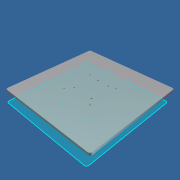
# Autodesk Inventor part: Acrylic_6_Base
Saved by Autodesk Inventor 2012 (Build 160160000, 160)
## iProperties
Created: 2014-03-30
Part Number: Acrylic_6_Base
Material: Default
Document SubType Name: Modeling
Designer: Admin
Density: 1 g/cm^3
Author: Admin
Autodesk Inventor part; units mm, degrees
ref_plane "YZ Plane" through (0, 0, 0) normal (1, 0, 0) x (0, 1, 0)
ref_plane "XZ Plane" through (0, 0, 0) normal (0, 1, 0) x (-1, 0, 0)
ref_plane "XY Plane" through (0, 0, 0) normal (0, 0, 1) x (1, 0, 0)
sketch "Sketch1" plane through (0, 0, 0) normal (0, 0, 1) x (1, 0, 0)
  line L0 (-162.4497, 0) -> (162.4497, 0) projected
  line L1 (0, -162.4497) -> (0, 162.4497) projected
  line L2 (-110, 115) -> (110, 115)
  line L3 (115, 110) -> (115, -110)
  line L4 (110, -115) -> (-110, -115)
  line L5 (-115, -110) -> (-115, 110)
  arc A0 (-110, 115) -> (-115, 110) centre (-110, 110) ccw
  arc A1 (115, 110) -> (110, 115) centre (110, 110) ccw
  arc A2 (110, -115) -> (115, -110) centre (110, -110) ccw
  arc A3 (-115, -110) -> (-110, -115) centre (-110, -110) ccw
  point P0 (0, 0)
  point P1 (115, -115)
  point P2 (115, 115)
  point P3 (-115, -115)
  dimension "d0" = 230
  dimension "d1" = 230
  dimension "d2" = 115
  dimension "d3" = 115
  dimension "d4" = 5
  constraints: 8 end point, 8 point on circle, 8 tangent, 6 point on line, 4 centre point, 3 equal radius, 2 parallel, 1 horizontal, 1 perpendicular
  measures "d0" distance of point (115, -115) point (-115, -115)
  measures "d1" distance of point (115, 115) point (115, -115)
  measures "d2" distance between parallel lines of L2 L0
  measures "d3" distance between parallel lines of L1 L5
  measures "d4" radius of A0
extrude "Extrusion1" add sketch "Sketch1" along normal blind 6
sketch "Sketch2" plane through (0, 0, 6) normal (0, 0, 1) x (1, 0, 0)
  circle A0 centre (-35.355, 35.355) radius 1.385
  circle A1 centre (-35.355, -35.355) radius 1.385
  circle A2 centre (35.355, -35.355) radius 1.385
  circle A3 centre (35.355, 35.355) radius 1.385
  circle A4 centre (-24.13, -19.01) radius 1.5875
  circle A5 centre (24.13, -20.28) radius 1.5875
  circle A6 centre (19.05, 31.79) radius 1.5875
  circle A7 centre (-8.89, 31.79) radius 1.5875
  point P0 (0, 0)
  constraints: 8 centre point, 16 other
extrude "Extrusion2" cut sketch "Sketch2" against normal through all
body "Solid1"
